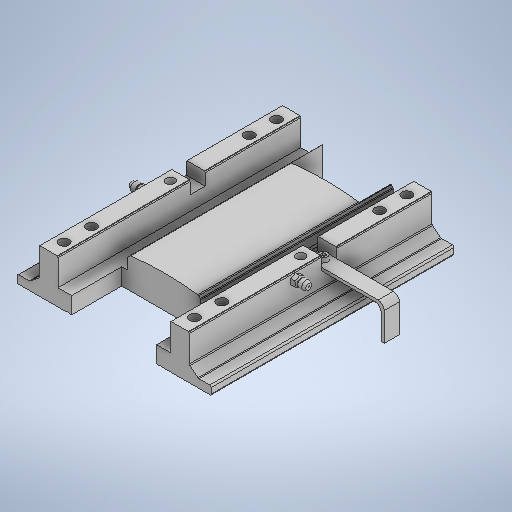
# Autodesk Inventor part: Mobile
Saved by Autodesk Inventor 2025.2 (Build 292293000, 293)
## iProperties
Category: PARTsolutions
Company: TOYO
Created: 2025-03-03
Part Number: Mobile
Material: Generic
Catalog Web Link: www.cadenas.de
Description: ETH2_17_4-ETH2
Vendor: TOYO
Document SubType Name: Modeling
Designer: psAdmin
Manufacturer: TOYO
Mass: 289.981 g
Surface Area: 627.917 cm^2
Volume: 289.981 cm^3
Density: 1 g/cm^3
Appearance: PSOLRGB-175-175-175
PSOL_IDENT_0: {$CADENAS_DATA/23d-libs/toyo/eth2_series/eth2_17/parts/eth2_17_body4.prj},165 {VTYP=3D},{NB=ETH2-17-
PSOL_IDENT_1: L_4},{LINA=ETH2-17-L},{NN=ETH2_17_4},{DATE=02.07.2024 05:59:00},{GEOMDATE=13.06.2024 03:24:00},{VERS
PSOL_IDENT_2: ION=},{LINEID=10},{WBVAR=SD},{WBNUMERIC=}  {NB=ETH2-17-L_4},{LINA=ETH2-17-L},{KT=DUMMY},{CNSORDERNO=
PSOL_IDENT_3: ETH2-17-L},{MODEL=ETH2-17},{SD=L}
NB: ETH2-17-L_4
NN: ETH2_17_4
NT: ETH2
NBSYN: $CNSORDERNO._4
LINA: ETH2-17-L
CATALOG: TOYO
MODEL: ETH2-17
SD: L: Left side of slide
SUPPLIER: TOYO
ARTICLENO: ETH2-17-L_4
BOMINFO: ETH2-17-L
CREATOR: CADENAS GmbH
Title: ETH2-17-L
Author: Cadenas PARTsolutions
Comments: ETH2
Autodesk Inventor part; units mm, degrees
sketch "__1" plane through (0, 0, 0) normal (0, 0, 1) x (1, 0, 0)
  arc A0 (-64, 0.8142) -> (-63.7071, 0.1071) centre (-63, 0.8142) ccw
  line L0 (-63.7071, 0.1071) -> (-63.6, 0)
  line L1 (-63.6, 0) -> (-31.414, 0)
  line L2 (-31.414, 0) -> (-31.207, 0.207)
  arc A1 (-29.634, 0) -> (-31.207, 0.207) centre (-30.4999, -0.5002) ccw
  line L3 (-29.634, 0) -> (29.634, 0)
  arc A2 (31.207, 0.207) -> (29.634, 0) centre (30.4999, -0.5002) ccw
  line L4 (31.207, 0.207) -> (31.414, 0)
  line L5 (31.414, 0) -> (63.6, 0)
  line L6 (63.6, 0) -> (63.7071, 0.1071)
  arc A3 (63.7071, 0.1071) -> (64, 0.8142) centre (63, 0.8142) ccw
  line L7 (64, 0.8142) -> (64, 4.5)
  arc A4 (64, 4.5) -> (63, 5.5) centre (63, 4.5) ccw
  line L8 (63, 5.5) -> (55.8478, 5.5)
  arc A5 (55.227, 5.716) -> (55.8478, 5.5) centre (55.8478, 6.5) ccw
  line L9 (55.227, 5.716) -> (49.8793, 9.9498)
  arc A6 (49.5, 10.7338) -> (49.8793, 9.9498) centre (50.5, 10.7338) ccw
  line L10 (49.5, 10.7338) -> (49.5, 28.0858)
  arc A7 (49.5, 28.0858) -> (49.2071, 28.7929) centre (48.5, 28.0858) ccw
  line L11 (49.2071, 28.7929) -> (49, 29)
  line L12 (49, 29) -> (37.5, 29)
  line L13 (37.5, 29) -> (37.2929, 28.7929)
  arc A8 (37.2929, 28.7929) -> (37, 28.0858) centre (38, 28.0858) ccw
  line L14 (37, 28.0858) -> (37, 11)
  line L15 (37, 11) -> (25, 11)
  arc A9 (24, 12) -> (25, 11) centre (25, 12) ccw
  line L16 (24, 12) -> (24, 17.971)
  arc A10 (24, 17.971) -> (23.7527, 18.6293) centre (23, 17.971) ccw
  line L17 (23.7527, 18.6293) -> (22.7636, 19.7603)
  arc A11 (22.7636, 19.7603) -> (22.137, 20.094) centre (22.0109, 19.102) ccw
  arc A12 (22.137, 20.094) -> (-22.137, 20.094) centre (0, -153.5002) ccw
  arc A13 (-22.137, 20.094) -> (-22.7636, 19.7603) centre (-22.0109, 19.102) ccw
  line L18 (-22.7636, 19.7603) -> (-23.7527, 18.6293)
  arc A14 (-23.7527, 18.6293) -> (-24, 17.971) centre (-23, 17.971) ccw
  line L19 (-24, 17.971) -> (-24, 12)
  arc A15 (-25, 11) -> (-24, 12) centre (-25, 12) ccw
  line L20 (-25, 11) -> (-37, 11)
  line L21 (-37, 11) -> (-37, 28.0858)
  arc A16 (-37, 28.0858) -> (-37.2929, 28.7929) centre (-38, 28.0858) ccw
  line L22 (-37.2929, 28.7929) -> (-37.5, 29)
  line L23 (-37.5, 29) -> (-49, 29)
  line L24 (-49, 29) -> (-49.2071, 28.7929)
  arc A17 (-49.2071, 28.7929) -> (-49.5, 28.0858) centre (-48.5, 28.0858) ccw
  line L25 (-49.5, 28.0858) -> (-49.5, 10.7338)
  arc A18 (-49.8793, 9.9498) -> (-49.5, 10.7338) centre (-50.5, 10.7338) ccw
  line L26 (-49.8793, 9.9498) -> (-55.227, 5.716)
  arc A19 (-55.8478, 5.5) -> (-55.227, 5.716) centre (-55.8478, 6.5) ccw
  line L27 (-55.8478, 5.5) -> (-63, 5.5)
  arc A20 (-63, 5.5) -> (-64, 4.5) centre (-63, 4.5) ccw
  line L28 (-64, 4.5) -> (-64, 0.8142)
  constraints: 58 end point, 42 point on circle, 21 centre point
extrude "Extrusion1" add sketch "__1" against normal blind 160
sketch "__2" plane through (0, 0, 0) normal (0, 1, 0) x (-1, 0, 0)
  line L0 (28, -33) -> (28, 0)
  line L1 (28, 0) -> (-28, 0)
  line L2 (-28, 0) -> (-28, -33)
  line L3 (-28, -33) -> (28, -33)
  constraints: 8 end point
extrude "Extrusion2" cut sketch "__2" along normal blind 29
sketch "__3" plane through (0, 0, 0) normal (0, 1, 0) x (-1, 0, 0)
  line L0 (22.5, -160) -> (22.5, -139)
  line L1 (22.5, -139) -> (-22.5, -139)
  line L2 (-22.5, -139) -> (-22.5, -160)
  line L3 (-22.5, -160) -> (22.5, -160)
  constraints: 8 end point
extrude "Extrusion3" cut sketch "__3" along normal blind 29
sketch "__4" plane through (0, 0, -10) normal (0, 0, 1) x (1, 0, 0)
  line L0 (43, 10) -> (43, 29)
  line L1 (43, 29) -> (46.3235, 29)
  line L2 (46.3235, 29) -> (46.3235, 11)
  line L3 (46.3235, 11) -> (47, 11)
  line L4 (47, 11) -> (43, 10)
  line L5 (43, 10) -> (43, 29)
  constraints: 12 end point
revolve "Revolution1" cut sketch "__4" angle 360 about axis through (43, 10, -10) along (0, -1, 0)
thread "Thread1" size "M8x1.25" class "6H" standard "ISO Metric profile" full length
sketch "Pattern_1_SKETCH_1" plane through (0, 0, -28) normal (0, 0, 1) x (1, 0, 0)
  line L0 (43, 10) -> (43, 29)
  line L1 (43, 29) -> (46.3235, 29)
  line L2 (46.3235, 29) -> (46.3235, 11)
  line L3 (46.3235, 11) -> (47, 11)
  line L4 (47, 11) -> (43, 10)
  line L5 (43, 10) -> (43, 29)
  constraints: 12 end point
sketch "Pattern_1_SKETCH_2" plane through (0, 0, -132) normal (0, 0, 1) x (1, 0, 0)
  line L0 (43, 10) -> (43, 29)
  line L1 (43, 29) -> (46.3235, 29)
  line L2 (46.3235, 29) -> (46.3235, 11)
  line L3 (46.3235, 11) -> (47, 11)
  line L4 (47, 11) -> (43, 10)
  line L5 (43, 10) -> (43, 29)
  constraints: 12 end point
sketch "Pattern_1_SKETCH_3" plane through (0, 0, -150) normal (0, 0, 1) x (1, 0, 0)
  line L0 (43, 10) -> (43, 29)
  line L1 (43, 29) -> (46.3235, 29)
  line L2 (46.3235, 29) -> (46.3235, 11)
  line L3 (46.3235, 11) -> (47, 11)
  line L4 (47, 11) -> (43, 10)
  line L5 (43, 10) -> (43, 29)
  constraints: 12 end point
sketch "Pattern_1_SKETCH_4" plane through (0, 0, -150) normal (0, 0, 1) x (1, 0, 0)
  line L0 (-43, 10) -> (-43, 29)
  line L1 (-43, 29) -> (-39.6765, 29)
  line L2 (-39.6765, 29) -> (-39.6765, 11)
  line L3 (-39.6765, 11) -> (-39, 11)
  line L4 (-39, 11) -> (-43, 10)
  line L5 (-43, 10) -> (-43, 29)
  constraints: 12 end point
sketch "Pattern_1_SKETCH_5" plane through (0, 0, -132) normal (0, 0, 1) x (1, 0, 0)
  line L0 (-43, 10) -> (-43, 29)
  line L1 (-43, 29) -> (-39.6765, 29)
  line L2 (-39.6765, 29) -> (-39.6765, 11)
  line L3 (-39.6765, 11) -> (-39, 11)
  line L4 (-39, 11) -> (-43, 10)
  line L5 (-43, 10) -> (-43, 29)
  constraints: 12 end point
sketch "Pattern_1_SKETCH_6" plane through (0, 0, -28) normal (0, 0, 1) x (1, 0, 0)
  line L0 (-43, 10) -> (-43, 29)
  line L1 (-43, 29) -> (-39.6765, 29)
  line L2 (-39.6765, 29) -> (-39.6765, 11)
  line L3 (-39.6765, 11) -> (-39, 11)
  line L4 (-39, 11) -> (-43, 10)
  line L5 (-43, 10) -> (-43, 29)
  constraints: 12 end point
sketch "Pattern_1_SKETCH_7" plane through (0, 0, -10) normal (0, 0, 1) x (1, 0, 0)
  line L0 (-43, 10) -> (-43, 29)
  line L1 (-43, 29) -> (-39.6765, 29)
  line L2 (-39.6765, 29) -> (-39.6765, 11)
  line L3 (-39.6765, 11) -> (-39, 11)
  line L4 (-39, 11) -> (-43, 10)
  line L5 (-43, 10) -> (-43, 29)
  constraints: 12 end point
revolve "Revolution2" cut sketch "Pattern_1_SKETCH_1" angle 360 about axis through (43, 10, -28) along (0, -1, 0)
thread "Thread2" size "M8x1.25" class "6H" standard "ISO Metric profile" full length
revolve "Revolution3" cut sketch "Pattern_1_SKETCH_2" angle 360 about axis through (43, 10, -132) along (0, -1, 0)
thread "Thread3" size "M8x1.25" class "6H" standard "ISO Metric profile" full length
revolve "Revolution4" cut sketch "Pattern_1_SKETCH_3" angle 360 about axis through (43, 10, -150) along (0, -1, 0)
thread "Thread4" size "M8x1.25" class "6H" standard "ISO Metric profile" full length
revolve "Revolution5" cut sketch "Pattern_1_SKETCH_4" angle 360 about axis through (-43, 10, -150) along (0, -1, 0)
thread "Thread5" size "M8x1.25" class "6H" standard "ISO Metric profile" full length
revolve "Revolution6" cut sketch "Pattern_1_SKETCH_5" angle 360 about axis through (-43, 10, -132) along (0, -1, 0)
thread "Thread6" size "M8x1.25" class "6H" standard "ISO Metric profile" full length
revolve "Revolution7" cut sketch "Pattern_1_SKETCH_6" angle 360 about axis through (-43, 10, -28) along (0, -1, 0)
thread "Thread7" size "M8x1.25" class "6H" standard "ISO Metric profile" full length
revolve "Revolution8" cut sketch "Pattern_1_SKETCH_7" angle 360 about axis through (-43, 10, -10) along (0, -1, 0)
thread "Thread8" size "M8x1.25" class "6H" standard "ISO Metric profile" full length
sketch "Sketch12" plane through (37.5, 29, 0) normal (0, 1, 0) x (1, 0, 0)
  point P0 (5.5, 80)
hole "Hole1" at (43, 29, -80) direction (0, -1, 0) diameter 6 depth 15
sketch "Sketch13" plane through (-49, 29, 0) normal (0, 1, 0) x (1, 0, 0)
  point P0 (6, 80)
hole "Hole2" at (-43, 29, -80) direction (0, -1, 0) diameter 6 depth 15
sketch "__8" plane through (0, 29, 0) normal (0, 1, 0) x (1, 0, 0)
  line L0 (37, 97) -> (37, 87)
  line L1 (37, 87) -> (49.5, 87)
  line L2 (49.5, 87) -> (49.5, 97)
  line L3 (49.5, 97) -> (37, 97)
  constraints: 8 end point
extrude "Extrusion4" cut sketch "__8" against normal blind 8.5
sketch "__9" plane through (0, 29, 0) normal (0, 1, 0) x (1, 0, 0)
  line L0 (-49.5, 97) -> (-49.5, 87)
  line L1 (-49.5, 87) -> (-37, 87)
  line L2 (-37, 87) -> (-37, 97)
  line L3 (-37, 97) -> (-49.5, 97)
  constraints: 8 end point
extrude "Extrusion5" cut sketch "__9" against normal blind 8.5
sketch "__11" plane through (0, 0, -92) normal (0, 0, 1) x (1, 0, 0)
  line L0 (41.5, 22.5) -> (41.5, 20.5)
  line L1 (41.5, 20.5) -> (85, 20.5)
  arc A0 (89, 16.5) -> (85, 20.5) centre (85, 16.5) ccw
  line L2 (89, 16.5) -> (89, -0.25)
  line L3 (89, -0.25) -> (91, -0.25)
  line L4 (91, -0.25) -> (91, 18.5)
  arc A1 (91, 18.5) -> (87, 22.5) centre (87, 18.5) ccw
  line L5 (87, 22.5) -> (41.5, 22.5)
  constraints: 12 end point, 4 point on circle, 2 centre point
extrude "Extrusion6" add sketch "__11" along normal mid plane 10
sketch "__13" plane through (41.5, 22.5, -97) normal (0, 1, 0) x (0, 0, 1)
  circle A0 centre (5, 4.5) radius 2.75
  constraints: 1 centre point
extrude "Extrusion7" add sketch "__13" along normal blind 3
sketch "__14" plane through (46, 25.5, -92) normal (0, 1, 0) x (0, 0, 1)
  line L0 (-1.4434, 0) -> (-0.7217, -1.25)
  line L1 (-0.7217, -1.25) -> (0.7217, -1.25)
  line L2 (0.7217, -1.25) -> (1.4434, 0)
  line L3 (1.4434, 0) -> (0.7217, 1.25)
  line L4 (0.7217, 1.25) -> (-0.7217, 1.25)
  line L5 (-0.7217, 1.25) -> (-1.4434, 0)
  constraints: 12 end point
extrude "Extrusion8" cut sketch "__14" against normal blind 1.3
sketch "__17" plane through (0, 0, -70) normal (0, 0, 1) x (1, 0, 0)
  line L0 (58.3, 24.25) -> (49.5, 24.25)
  line L1 (49.5, 27.75) -> (49.5, 24.75)
  line L2 (49.5, 24.75) -> (58.3, 24.75)
  line L3 (58.3, 24.75) -> (58.3, 26.21)
  line L4 (58.3, 26.21) -> (56.43, 27.1)
  arc A0 (56.43, 27.1) -> (53.5824, 26.84) centre (55.3459, 23.2497) ccw
  arc A1 (53.19, 26.8192) -> (53.5824, 26.84) centre (53.362, 27.2887) ccw
  arc A2 (51.99, 27.75) -> (53.19, 26.8192) centre (54.0498, 29.1667) ccw
  line L5 (51.99, 27.75) -> (49.5, 27.75)
  constraints: 12 end point, 6 point on circle, 3 centre point
revolve "Revolution9" add sketch "__17" angle 360 about axis through (58.3, 24.25, -70) along (1, 0, 0)
sketch "__18" plane through (58.3, 24.25, -70) normal (1, 0, 0) x (0, 1, 0)
  circle A0 centre (0, 0) radius 5
  line L0 (-3.4641, 0) -> (-1.7321, -3)
  line L1 (-1.7321, -3) -> (1.7321, -3)
  line L2 (1.7321, -3) -> (3.4641, 0)
  line L3 (3.4641, 0) -> (1.7321, 3)
  line L4 (1.7321, 3) -> (-1.7321, 3)
  line L5 (-1.7321, 3) -> (-3.4641, 0)
  constraints: 12 end point, 1 centre point
extrude "Extrusion9" cut sketch "__18" against normal blind 8.8
sketch "__21" plane through (0, 0, -70) normal (0, 0, 1) x (1, 0, 0)
  line L0 (-49.5, 24.25) -> (-58.3, 24.25)
  line L1 (-58.3, 26.21) -> (-58.3, 24.75)
  line L2 (-58.3, 24.75) -> (-49.5, 24.75)
  line L3 (-49.5, 24.75) -> (-49.5, 27.75)
  line L4 (-49.5, 27.75) -> (-51.99, 27.75)
  arc A0 (-53.19, 26.8192) -> (-51.99, 27.75) centre (-54.0498, 29.1667) ccw
  arc A1 (-53.5824, 26.84) -> (-53.19, 26.8192) centre (-53.362, 27.2887) ccw
  arc A2 (-53.5824, 26.84) -> (-56.43, 27.1) centre (-55.3459, 23.2497) ccw
  line L5 (-56.43, 27.1) -> (-58.3, 26.21)
  constraints: 12 end point, 6 point on circle, 3 centre point
revolve "Revolution10" add sketch "__21" angle 360 about axis through (-49.5, 24.25, -70) along (1, 0, 0)
sketch "__19" plane through (-58.3, 24.25, -70) normal (-1, 0, 0) x (0, 1, 0)
  circle A0 centre (0, 0) radius 5
  line L0 (-3.4641, 0) -> (-1.7321, -3)
  line L1 (-1.7321, -3) -> (1.7321, -3)
  line L2 (1.7321, -3) -> (3.4641, 0)
  line L3 (3.4641, 0) -> (1.7321, 3)
  line L4 (1.7321, 3) -> (-1.7321, 3)
  line L5 (-1.7321, 3) -> (-3.4641, 0)
  constraints: 12 end point, 1 centre point
extrude "Extrusion10" cut sketch "__19" against normal blind 8.8
ref_plane "BODY4_XY" through (0, 0, -80) normal (0, 0, -1) x (1, 0, 0)
ref_plane "BODY4_YZ" through (0, 0, -80) normal (1, 0, 0) x (0, -1, 0)
ref_plane "BODY4_ZX" through (0, 0, -80) normal (0, -1, 0) x (0, 0, -1)
body "Solid1"
